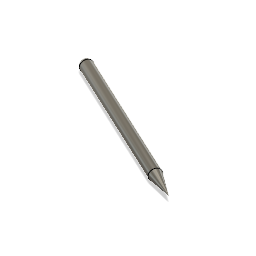
铅笔 (Autodesk Fusion 360 design; units mm, degrees)
Autodesk Fusion 360 part; units mm, degrees
cylinder "圆柱体基本要素1" add diameter 8 height 100 placed x (1, 0, 0) y (0, 1, 0) z (0, 0, 1) at (0, 0, 0) makes body 1
sphere "球体基本要素1" add diameter 8 placed x (1, 0, 0) y (0, 1, 0) z (0, 0, 1) at (0, 0, 0) bodies 1
sketch "草图3" plane through (0, 0, 0) normal (0, 0, 1) x (1, 0, 0)
  line L0 (-230, 90) -> (-230, 70)
  line L1 (-230, 70) -> (-226, 70)
  line L2 (-230, 90) -> (-226, 70)
  dimension "d5" = 4
revolve "旋转1" add sketch "草图3" angle 360 about axis through (-230, 90, 0) along (0, -1, 0) separate body makes body 2
move_body "移动1" bodies 2 to x (1, 0, 0) y (0, 0, 1) z (0, -1, 0) at (171.3611, -87.8678, -75.1672)
move_body "移动2" bodies 2 to x (-0.422618, 0, 0.906308) y (0, 1, 0) z (-0.906308, 0, -0.422618) at (-109.0099, 22.8921, 43.7626)
move_body "对齐1" bodies 1 to x (0.422618, 0, -0.906308) y (0, 1, 0) z (0.906308, 0, 0.422618) at (-197.0279, 0, 8.1244)
move_body "移动3" bodies 2 to x (-1, 0, 0) y (0, 1, 0) z (0, 0, -1) at (-175.6009, 0, 49.9387)
move_body "移动4" bodies 2 to x (1, 0, 0) y (0, 1, 0) z (0, 0, 1) at (0, 70, 0)
move_body "对齐2" bodies 2 to x (1, 0, 0) y (0, 1, 0) z (0, 0, 1) at (0.7388, -5.0243, -1.5843)
move_body "移动5" bodies 2 to x (1, 0, 0) y (0, 1, 0) z (0, 0, 1) at (-11.0303, 0, -5.1215)
combine "合并1" operation add target body 2 tool bodies 1 makes body 3 at (-165.1293, -0.1994, 18.5909)
